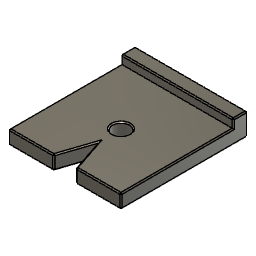
guide-10mm-edge-plate v3 (Autodesk Fusion 360 design; units mm, degrees)
Autodesk Fusion 360 part; units mm, degrees
sketch "Sketch1" plane through (0, 0, 0) normal (0, 1, 0) x (1, 0, 0)
  line L0 (-10, 0) -> (10, 0)
  line L1 (10, 0) -> (10, -20)
  line L2 (-10, -20) -> (-10, 0)
  circle A0 centre (0, -10) radius 1.5
  line L3 (-2, -20) -> (0, -14)
  line L4 (0, -14) -> (2, -20)
  line L5 (-10, -20) -> (-2, -20)
  line L6 (2, -20) -> (10, -20)
  dimension "d1" = 3
  dimension "d2" = 20
  dimension "d3" = 20
  dimension "d4" = 10
  dimension "d11" = 4
  dimension "d12" = 2
  dimension "d13" = 4
  dimension "d14" = 10
  constraint horizontal L0
  constraint vertical L1
  constraint vertical L2
  constraint collinear origin L0.start L0.end
  constraint horizontal L5
  constraint perpendicular L1 L6
  constraint vertical A0.centre L3.end
  constraint vertical origin A0.centre
  constraint horizontal L3.start L4.end
  measures "d1" diameter of A0
  measures "d2" distance of L0.end L1.end
  measures "d3" distance of L1.end L2.start
  measures "d4" distance of origin L0.start
  measures "d11" distance of L3.start L4.end
  measures "d12" horizontal distance of A0.centre L3.start
  measures "d13" distance of A0.centre L3.end
  measures "d14" distance of origin A0.centre
extrude "Extrude1" add sketch "Sketch1" along normal blind 2.5
sketch "Sketch2" plane through (0, 0, 0) normal (0, 0, -1) x (-1, 0, 0)
  line L0 (-10, 0) -> (10, 0)
  line L1 (10, 0) -> (10, 2.5)
  line L2 (10, 2.5) -> (-10, 2.5)
  line L3 (-10, 2.5) -> (-10, 0)
  line L4 (-10, 0) -> (10, 0)
  line L5 (10, 0) -> (10, 4)
  line L6 (10, 4) -> (-10, 4)
  line L7 (-10, 4) -> (-10, 0)
  dimension "d7" = 1.5
  constraint horizontal L4
  constraint vertical L5
  constraint horizontal L6
  constraint vertical L7
  constraint coincident L0.start L3.end
  constraint coincident L0.end L1.start
  measures "d7" distance of L2.end L6.end
extrude "Extrude2" add sketch "Sketch2" along normal blind 2.5
chamfer "Chamfer2" distance 0.2 angle 45 27 edges at (1, 0, 17) (-1, 0, 17) (-2, 1.25, 20) (2, 1.25, 20) (6, 0, 20) (10, 1.25, 20) (10, 0, 8.75) (-6, 0, 20) (-10, 1.25, 20) (-6, 2.5, 20) (6, 2.5, 20) (10, 2.5, 10) (10, 3.25, 0) (10, 4, -1.25) (10, 2, -2.5) (0, 0, -2.5) (-10, 0, 8.75) (-1.3985, 0, 9.4576) (0, 4, -2.5) (0, 4, 0) (-10, 4, -1.25) (-10, 2.5, 10) (-10, 3.25, 0) (-10, 2, -2.5) (1, 2.5, 17) (-1, 2.5, 17) (-1.3985, 2.5, 9.4576)
